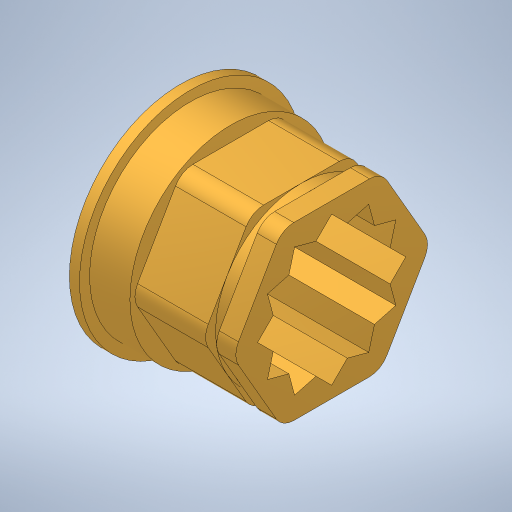
# Autodesk Inventor part: Bushing
Saved by Autodesk Inventor 2023.2 (Build 272271000, 271)
## iProperties
Created: 2024-01-10
Part Number: Bushing
Material: Brass, Soft Yellow
Document SubType Name: Modeling
Designer: Nathan Cai
Mass: 18.4259 g
Surface Area: 22.2269 cm^2
Volume: 2.17543 cm^3
Density: 8.47 g/cm^3
Appearance: Brass - Satin
Author: Nathan Cai
Autodesk Inventor part; units mm, degrees
ref_plane "YZ Plane" through (0, 0, 0) normal (1, 0, 0) x (0, 1, 0)
ref_plane "XZ Plane" through (0, 0, 0) normal (0, 1, 0) x (-1, 0, 0)
ref_plane "XY Plane" through (0, 0, 0) normal (0, 0, 1) x (1, 0, 0)
sketch "Sketch1" plane through (0, 0, 0) normal (1, 0, 0) x (0, 1, 0)
  circle A0 centre (0, 0) radius 6 construction
  line L0 (6, 0) -> (0, 0) construction
  line L1 (4.2426, 0) -> (5.7956, 1.5529) construction
  line L2 (5.7956, 1.5529) -> (7.3485, 0)
  line L3 (7.3485, 0) -> (5.7956, -1.5529)
  line L4 (5.7956, -1.5529) -> (4.2426, 0) construction
  line L5 (3.6742, 2.1213) -> (4.2426, 4.2426) construction
  line L6 (4.2426, 4.2426) -> (6.364, 3.6742)
  line L7 (6.364, 3.6742) -> (5.7956, 1.5529)
  line L8 (5.7956, 1.5529) -> (3.6742, 2.1213) construction
  line L9 (2.1213, 3.6742) -> (1.5529, 5.7956) construction
  line L10 (1.5529, 5.7956) -> (3.6742, 6.364)
  line L11 (3.6742, 6.364) -> (4.2426, 4.2426)
  line L12 (4.2426, 4.2426) -> (2.1213, 3.6742) construction
  line L13 (0, 4.2426) -> (-1.5529, 5.7956) construction
  line L14 (-1.5529, 5.7956) -> (0, 7.3485)
  line L15 (0, 7.3485) -> (1.5529, 5.7956)
  line L16 (1.5529, 5.7956) -> (0, 4.2426) construction
  line L17 (-2.1213, 3.6742) -> (-4.2426, 4.2426) construction
  line L18 (-4.2426, 4.2426) -> (-3.6742, 6.364)
  line L19 (-3.6742, 6.364) -> (-1.5529, 5.7956)
  line L20 (-1.5529, 5.7956) -> (-2.1213, 3.6742) construction
  line L21 (-3.6742, 2.1213) -> (-5.7956, 1.5529) construction
  line L22 (-5.7956, 1.5529) -> (-6.364, 3.6742)
  line L23 (-6.364, 3.6742) -> (-4.2426, 4.2426)
  line L24 (-4.2426, 4.2426) -> (-3.6742, 2.1213) construction
  line L25 (-4.2426, 0) -> (-5.7956, -1.5529) construction
  line L26 (-5.7956, -1.5529) -> (-7.3485, 0)
  line L27 (-7.3485, 0) -> (-5.7956, 1.5529)
  line L28 (-5.7956, 1.5529) -> (-4.2426, 0) construction
  line L29 (-3.6742, -2.1213) -> (-4.2426, -4.2426) construction
  line L30 (-4.2426, -4.2426) -> (-6.364, -3.6742)
  line L31 (-6.364, -3.6742) -> (-5.7956, -1.5529)
  line L32 (-5.7956, -1.5529) -> (-3.6742, -2.1213) construction
  line L33 (-2.1213, -3.6742) -> (-1.5529, -5.7956) construction
  line L34 (-1.5529, -5.7956) -> (-3.6742, -6.364)
  line L35 (-3.6742, -6.364) -> (-4.2426, -4.2426)
  line L36 (-4.2426, -4.2426) -> (-2.1213, -3.6742) construction
  line L37 (0, -4.2426) -> (1.5529, -5.7956) construction
  line L38 (1.5529, -5.7956) -> (0, -7.3485)
  line L39 (0, -7.3485) -> (-1.5529, -5.7956)
  line L40 (-1.5529, -5.7956) -> (0, -4.2426) construction
  line L41 (2.1213, -3.6742) -> (4.2426, -4.2426) construction
  line L42 (4.2426, -4.2426) -> (3.6742, -6.364)
  line L43 (3.6742, -6.364) -> (1.5529, -5.7956)
  line L44 (1.5529, -5.7956) -> (2.1213, -3.6742) construction
  line L45 (3.6742, -2.1213) -> (5.7956, -1.5529) construction
  line L46 (5.7956, -1.5529) -> (6.364, -3.6742)
  line L47 (6.364, -3.6742) -> (4.2426, -4.2426)
  line L48 (4.2426, -4.2426) -> (3.6742, -2.1213) construction
  circle A1 centre (0, 0) radius 8.5 construction
  line L49 (8.5, -4.9075) -> (0, -9.815)
  line L50 (0, -9.815) -> (-8.5, -4.9075)
  line L51 (-8.5, -4.9075) -> (-8.5, 4.9075)
  line L52 (-8.5, 4.9075) -> (0, 9.815)
  line L53 (0, 9.815) -> (8.5, 4.9075)
  line L54 (8.5, 4.9075) -> (8.5, -4.9075)
  point P0 (5.7956, 0)
  point P1 (5.1962, 3)
  point P2 (5.0191, 2.8978)
  point P3 (3, 5.1962)
  point P4 (2.8978, 5.0191)
  point P5 (0, 6)
  point P6 (0, 5.7956)
  point P7 (-3, 5.1962)
  point P8 (-2.8978, 5.0191)
  point P9 (-5.1962, 3)
  point P10 (-5.0191, 2.8978)
  point P11 (-6, 0)
  point P12 (-5.7956, 0)
  point P13 (-5.1962, -3)
  point P14 (-5.0191, -2.8978)
  point P15 (-3, -5.1962)
  point P16 (-2.8978, -5.0191)
  point P17 (0, -6)
  point P18 (0, -5.7956)
  point P19 (3, -5.1962)
  point P20 (2.8978, -5.0191)
  point P21 (5.1962, -3)
  point P22 (5.0191, -2.8978)
  point P23 (8.5, 0)
  dimension "d0" = 12
  dimension "d3" = 360
  dimension "d5" = 17
  constraints: 110 end point, 4 coincident, 3 point on line, 2 centre point, 2 point on circle, 1 horizontal, 1 midpoint, 1 tangent, 143 other
  measures "d0" diameter of A0
  measures "d5" diameter of A1
extrude "Extrusion1" add sketch "Sketch1" along normal blind 15
sketch "Sketch2" plane through (0, 0, 0) normal (-1, 0, 0) x (0, 0, 1)
  circle A0 centre (0, 0) radius 10
  line L0 (1.5529, 5.7956) -> (0, 7.3485) projected
  line L1 (3.6742, 6.364) -> (1.5529, 5.7956) projected
  line L2 (4.2426, 4.2426) -> (3.6742, 6.364) projected
  line L3 (6.364, 3.6742) -> (4.2426, 4.2426) projected
  line L4 (5.7956, 1.5529) -> (6.364, 3.6742) projected
  line L5 (7.3485, 0) -> (5.7956, 1.5529) projected
  line L6 (5.7956, -1.5529) -> (7.3485, 0) projected
  line L7 (6.364, -3.6742) -> (5.7956, -1.5529) projected
  line L8 (4.2426, -4.2426) -> (6.364, -3.6742) projected
  line L9 (3.6742, -6.364) -> (4.2426, -4.2426) projected
  line L10 (1.5529, -5.7956) -> (3.6742, -6.364) projected
  line L11 (0, -7.3485) -> (1.5529, -5.7956) projected
  line L12 (-1.5529, -5.7956) -> (0, -7.3485) projected
  line L13 (-3.6742, -6.364) -> (-1.5529, -5.7956) projected
  line L14 (-4.2426, -4.2426) -> (-3.6742, -6.364) projected
  line L15 (-6.364, -3.6742) -> (-4.2426, -4.2426) projected
  line L16 (-5.7956, -1.5529) -> (-6.364, -3.6742) projected
  line L17 (-7.3485, 0) -> (-5.7956, -1.5529) projected
  line L18 (-5.7956, 1.5529) -> (-7.3485, 0) projected
  line L19 (-6.364, 3.6742) -> (-5.7956, 1.5529) projected
  line L20 (-4.2426, 4.2426) -> (-6.364, 3.6742) projected
  line L21 (-3.6742, 6.364) -> (-4.2426, 4.2426) projected
  line L22 (-1.5529, 5.7956) -> (-3.6742, 6.364) projected
  line L23 (0, 7.3485) -> (-1.5529, 5.7956) projected
  line L24 (0, 7.3485) -> (-1.5529, 5.7956) projected
  line L25 (4.9075, 8.5) -> (9.815, 0) projected
  line L26 (-4.9075, 8.5) -> (4.9075, 8.5) projected
  line L27 (-9.815, 0) -> (-4.9075, 8.5) projected
  line L28 (-4.9075, -8.5) -> (-9.815, 0) projected
  line L29 (4.9075, -8.5) -> (-4.9075, -8.5) projected
  line L30 (9.815, 0) -> (4.9075, -8.5) projected
  line L31 (1.5529, 5.7956) -> (0, 7.3485) projected
  line L32 (3.6742, 6.364) -> (1.5529, 5.7956) projected
  line L33 (4.2426, 4.2426) -> (3.6742, 6.364) projected
  line L34 (6.364, 3.6742) -> (4.2426, 4.2426) projected
  line L35 (5.7956, 1.5529) -> (6.364, 3.6742) projected
  line L36 (7.3485, 0) -> (5.7956, 1.5529) projected
  line L37 (5.7956, -1.5529) -> (7.3485, 0) projected
  line L38 (6.364, -3.6742) -> (5.7956, -1.5529) projected
  line L39 (4.2426, -4.2426) -> (6.364, -3.6742) projected
  line L40 (3.6742, -6.364) -> (4.2426, -4.2426) projected
  line L41 (1.5529, -5.7956) -> (3.6742, -6.364) projected
  line L42 (0, -7.3485) -> (1.5529, -5.7956) projected
  line L43 (-1.5529, -5.7956) -> (0, -7.3485) projected
  line L44 (-3.6742, -6.364) -> (-1.5529, -5.7956) projected
  line L45 (-4.2426, -4.2426) -> (-3.6742, -6.364) projected
  line L46 (-6.364, -3.6742) -> (-4.2426, -4.2426) projected
  line L47 (-5.7956, -1.5529) -> (-6.364, -3.6742) projected
  line L48 (-7.3485, 0) -> (-5.7956, -1.5529) projected
  line L49 (-5.7956, 1.5529) -> (-7.3485, 0) projected
  line L50 (-6.364, 3.6742) -> (-5.7956, 1.5529) projected
  line L51 (-4.2426, 4.2426) -> (-6.364, 3.6742) projected
  line L52 (-3.6742, 6.364) -> (-4.2426, 4.2426) projected
  line L53 (-1.5529, 5.7956) -> (-3.6742, 6.364) projected
  line L54 (0, 7.3485) -> (-1.5529, 5.7956) projected
  circle A1 centre (0, 0) radius 8.5 construction
  line L55 (-4.9075, 8.5) -> (4.9075, 8.5) projected
  line L56 (-4.9075, -8.5) -> (-9.815, 0) projected
  line L57 (9.815, 0) -> (4.9075, -8.5) projected
  point P0 (0, 0)
  dimension "d12" = 1.5
  constraints: 3 tangent, 2 centre point, 1 coincident
  measures "d12" radial gap between concentric circles of A1 A0
extrude "Extrusion2" add sketch "Sketch2" against normal blind 5 contours A0 | L25 L30 L29 L28 L27 L26
fillet "Fillet1" radius 2 6 edges at (10, 8.5, 4.9075) (10, 8.5, -4.9075) (10, 0, 9.815) (10, -8.5, 4.9075) (10, -8.5, -4.9075) (10, 0, -9.815)
ref_plane "Work Plane1" through (9, 0, 0) normal (1, 0, 0) x (0, 0, -1)
sketch "Sketch4" plane through (0, 0, 0) normal (-1, 0, 0) x (0, 0, 1)
  circle A0 centre (0, 0) radius 10 projected
  line L0 (1.5529, 5.7956) -> (0, 7.3485) projected
  line L1 (3.6742, 6.364) -> (1.5529, 5.7956) projected
  line L2 (4.2426, 4.2426) -> (3.6742, 6.364) projected
  line L3 (6.364, 3.6742) -> (4.2426, 4.2426) projected
  line L4 (5.7956, 1.5529) -> (6.364, 3.6742) projected
  line L5 (7.3485, 0) -> (5.7956, 1.5529) projected
  line L6 (5.7956, -1.5529) -> (7.3485, 0) projected
  line L7 (6.364, -3.6742) -> (5.7956, -1.5529) projected
  line L8 (4.2426, -4.2426) -> (6.364, -3.6742) projected
  line L9 (3.6742, -6.364) -> (4.2426, -4.2426) projected
  line L10 (1.5529, -5.7956) -> (3.6742, -6.364) projected
  line L11 (0, -7.3485) -> (1.5529, -5.7956) projected
  line L12 (-1.5529, -5.7956) -> (0, -7.3485) projected
  line L13 (-3.6742, -6.364) -> (-1.5529, -5.7956) projected
  line L14 (-4.2426, -4.2426) -> (-3.6742, -6.364) projected
  line L15 (-6.364, -3.6742) -> (-4.2426, -4.2426) projected
  line L16 (-5.7956, -1.5529) -> (-6.364, -3.6742) projected
  line L17 (-7.3485, 0) -> (-5.7956, -1.5529) projected
  line L18 (-5.7956, 1.5529) -> (-7.3485, 0) projected
  line L19 (-6.364, 3.6742) -> (-5.7956, 1.5529) projected
  line L20 (-4.2426, 4.2426) -> (-6.364, 3.6742) projected
  line L21 (-3.6742, 6.364) -> (-4.2426, 4.2426) projected
  line L22 (-1.5529, 5.7956) -> (-3.6742, 6.364) projected
  line L23 (0, 7.3485) -> (-1.5529, 5.7956) projected
  circle A1 centre (0, 0) radius 11
  point P0 (0, 0)
  dimension "d20" = 1
  constraints: 1 centre point
  measures "d20" radial gap between concentric circles of A0 A1
extrude "Extrusion4" add sketch "Sketch4" against normal blind 1 contours A1
ref_plane "Work Plane2" through (12, 0, 0) normal (1, 0, 0) x (0, 0, -1)
sketch "Sketch5" plane through (12, 0, 0) normal (1, 0, 0) x (0, 0, -1)
  circle A0 centre (0, 0) radius 8.5
  circle A1 centre (0, 0) radius 12.5
  dimension "d24" = 17
  dimension "d25" = 25
  constraints: 2 centre point, 2 coincident
  measures "d24" diameter of A0
  measures "d25" diameter of A1
extrude "Extrusion5" cut sketch "Sketch5" along normal blind 1.1
body "Solid1"
